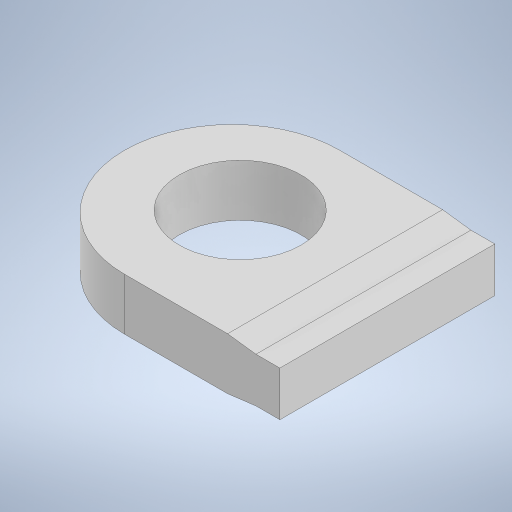
# Autodesk Inventor part: fan
Saved by Autodesk Inventor 2024 (Build 280153000, 153)
## iProperties
Created: 2024-10-17
Part Number: fan
Material: Generic
Document SubType Name: Modeling
Designer: Owner
Density: 1 g/cm^3
Appearance: Default
Author: Owner
Autodesk Inventor part; units mm, degrees
ref_plane "YZ Plane" through (0, 0, 0) normal (1, 0, 0) x (0, 1, 0)
ref_plane "XZ Plane" through (0, 0, 0) normal (0, 1, 0) x (-1, 0, 0)
ref_plane "XY Plane" through (0, 0, 0) normal (0, 0, 1) x (1, 0, 0)
sketch "Sketch1" plane through (0, 0, 0) normal (0, 1, 0) x (-1, 0, 0)
  line L0 (-55.88, 45.72) -> (55.88, 45.72)
  line L1 (55.88, 45.72) -> (55.88, -45.72)
  line L2 (55.88, -45.72) -> (-55.88, -45.72)
  line L3 (-55.88, -45.72) -> (-55.88, 45.72)
  line L4 (-55.88, 45.72) -> (55.88, -45.72) construction
  line L5 (55.88, 45.72) -> (-55.88, -45.72) construction
  circle A0 centre (10.16, 0) radius 45.72
  point P0 (0, 0)
  point P1 (10.16, -45.72)
  point P2 (10.16, 45.72)
  dimension "d0" = 111.76
  dimension "d1" = 91.44
  constraints: 12 end point, 3 tangent, 2 midpoint, 2 parallel, 1 centre point, 1 horizontal, 1 perpendicular
  measures "d0" distance of L1.end L2.end
  measures "d1" distance of L0.end L1.end
extrude "Extrusion1" add sketch "Sketch1" along normal blind 22.098 contours L0 A0 L2 L3 | A0
sketch "Sketch2" plane through (55.88, 0, -45.72) normal (0, 0, -1) x (-1, 0, 0)
  line L0 (66.04, 22.098) -> (0, 22.098) projected
  line L1 (66.04, 0) -> (0, 0) projected
  line L2 (0, 22.098) -> (10.16, 22.098)
  line L3 (10.16, 22.098) -> (10.16, 0)
  line L4 (10.16, 0) -> (0, 0)
  line L5 (0, 0) -> (0, 22.098)
  line L6 (5.08, 22.098) -> (5.08, 0)
  line L7 (0, 11.049) -> (10.16, 11.049)
  line L8 (0, 20.574) -> (10.16, 20.574)
  line L9 (10.16, 20.574) -> (10.16, 1.524)
  line L10 (10.16, 1.524) -> (0, 1.524)
  line L11 (0, 1.524) -> (0, 20.574)
  line L12 (0, 20.574) -> (10.16, 1.524) construction
  line L13 (10.16, 20.574) -> (0, 1.524) construction
  line L14 (10.16, 22.098) -> (22.225, 22.098)
  line L15 (22.225, 22.098) -> (22.225, 0)
  line L16 (22.225, 0) -> (10.16, 0)
  line L17 (10.16, 0) -> (10.16, 22.098)
  line L18 (10.16, 20.574) -> (22.225, 22.098)
  line L19 (22.225, 0) -> (10.16, 1.524)
  line L20 (5.08, 1.524) -> (10.16, 1.524)
  line L21 (5.08, 20.574) -> (10.16, 20.574)
  point P0 (55.88, 0)
  point P1 (5.08, 11.049)
  dimension "d4" = 10.16
  dimension "d5" = 19.05
  dimension "d6" = 12.065
  constraints: 40 end point, 9 midpoint, 6 parallel, 5 point on line, 4 perpendicular, 3 horizontal, 1 collinear
  measures "d4" distance of L3.end L4.end
  measures "d5" distance of L8.end L9.end
  measures "d6" distance of L15.end L16.end
extrude "Extrusion2" cut sketch "Sketch2" against normal blind 254 contours L18 L3 L0 | L3 L8 L6 L0 | L1 L3 L19 | L6 L8 L5 L0 | L1 L6 L10 L3 | L1 L5 L10 L6
sketch "Sketch3" plane through (0, 22.098, 0) normal (0, 1, 0) x (1, 0, 0)
  line L0 (-10.16, -45.72) -> (33.655, -45.72) projected
  line L1 (33.655, -45.72) -> (33.655, -23.368)
  line L2 (33.655, 45.72) -> (33.655, -45.72) projected
  line L3 (33.655, -23.368) -> (-49.457, -23.368)
  arc A0 (-10.16, 45.72) -> (-10.16, -45.72) centre (-10.16, 0) ccw projected
  line L4 (45.72, 45.72) -> (33.655, 45.72) projected
  line L5 (33.655, 45.72) -> (33.655, 28.448)
  line L6 (33.655, 28.448) -> (-45.9515, 28.448)
  line L7 (55.88, -45.72) -> (55.88, 45.72) projected
  line L8 (55.88, 28.448) -> (16.637, 28.448)
  line L9 (16.637, 28.448) -> (16.637, -23.368)
  circle A1 centre (-9.271, 2.54) radius 25.908
  point P0 (0, 0)
  dimension "d9" = 22.352
  dimension "d10" = 17.272
  dimension "d11" = 39.243
  constraints: 12 end point, 6 point on line, 3 perpendicular, 3 tangent, 2 point on circle, 1 centre point
  measures "d9" distance of L0.end L1.end
  measures "d10" distance of L2.start L5.end
  measures "d11" distance of L8.start L8.end
extrude "Extrusion3" cut sketch "Sketch3" against normal blind 254 contours A1
body "Solid1"
